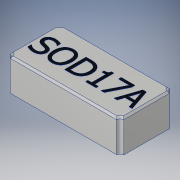
# Autodesk Inventor part: Crystal_ECX-34
Saved by Autodesk Inventor 2018 (Build 220112000, 112)
## iProperties
Created: 2016-08-15
Part Number: Crystal_ECX-34
Material: Aluminum 6061
Document SubType Name: Modeling
Designer: Bradley
Density: 2.7 g/cm^3
Appearance: Aluminum - Flat
Author: Bradley
Autodesk Inventor part; units mm, degrees
ref_plane "YZ Plane" through (0, 0, 0) normal (1, 0, 0) x (0, 1, 0)
ref_plane "XZ Plane" through (0, 0, 0) normal (0, 1, 0) x (-1, 0, 0)
ref_plane "XY Plane" through (0, 0, 0) normal (0, 0, 1) x (1, 0, 0)
sketch "Sketch1" plane through (0, 0, 0) normal (0, 1, 0) x (-1, 0, 0)
  line L0 (-1.6, 0.75) -> (1.6, 0.75)
  line L1 (1.6, 0.75) -> (1.6, -0.75)
  line L2 (1.6, -0.75) -> (-1.6, -0.75)
  line L3 (-1.6, -0.75) -> (-1.6, 0.75)
  line L4 (-1.6, 0.75) -> (1.6, -0.75) construction
  line L5 (1.6, 0.75) -> (-1.6, -0.75) construction
  arc A0 (1.6, -0.65) -> (1.5, -0.75) centre (1.6, -0.75) ccw
  arc A1 (-1.5, -0.75) -> (-1.6, -0.65) centre (-1.6, -0.75) ccw
  arc A2 (-1.6, 0.65) -> (-1.5, 0.75) centre (-1.6, 0.75) ccw
  arc A3 (1.5, 0.75) -> (1.6, 0.65) centre (1.6, 0.75) ccw
  point P0 (0, 0)
  dimension "d0" = 3.2
  dimension "d1" = 1.5
  dimension "d4" = 0.1
  constraints: 12 end point, 8 point on circle, 8 point on line, 4 centre point, 4 coincident, 3 equal radius, 2 midpoint, 2 parallel, 1 horizontal, 1 perpendicular
  measures "d0" distance of L1.end L2.end
  measures "d1" distance of L0.end L1.end
  measures "d4" radius of A0
extrude "Extrusion1" add sketch "Sketch1" along normal mid plane 0.9 contours L0 A3 L1 A0 L2 A1 L3 A2
chamfer "Chamfer1" distance 0.05 angle 45 8 edges at (0, 0.45, 0.75) (-1.5293, 0.45, 0.6793) (-1.6, 0.45, 0) (-1.5293, 0.45, -0.6793) (0, 0.45, -0.75) (1.5293, 0.45, -0.6793) (1.6, 0.45, 0) (1.5293, 0.45, 0.6793)
sketch "Sketch2" plane through (0, -0.45, 0) normal (0, -1, 0) x (1, 0, 0)
  line L0 (-1.6, 0.65) -> (-1.6, -0.65) projected
  arc A0 (-1.5, -0.75) -> (-1.6, -0.65) centre (-1.6, -0.75) ccw projected
  line L1 (-1.5, -0.75) -> (1.5, -0.75) projected
  arc A1 (1.6, -0.65) -> (1.5, -0.75) centre (1.6, -0.75) ccw projected
  line L2 (1.6, -0.65) -> (1.6, 0.65) projected
  arc A2 (1.5, 0.75) -> (1.6, 0.65) centre (1.6, 0.75) ccw projected
  line L3 (1.5, 0.75) -> (-1.5, 0.75) projected
  arc A3 (-1.6, 0.65) -> (-1.5, 0.75) centre (-1.6, 0.75) ccw projected
  arc A4 (-1.5, -0.75) -> (-1.6, -0.65) centre (-1.6, -0.75) ccw projected
  line L4 (-1.5741, -0.6534) -> (-1.5034, -0.5827)
  line L5 (-1.5034, -0.5827) -> (-1.5034, 0.5827)
  line L6 (-1.5034, 0.5827) -> (-1.5741, 0.6534)
  arc A5 (-1.6, 0.65) -> (-1.5, 0.75) centre (-1.6, 0.75) ccw projected
  line L7 (-1.5034, 0.7241) -> (-1.4327, 0.6534)
  line L8 (-1.4327, 0.6534) -> (-1.2, 0.6534)
  line L9 (-1.2, 0.6534) -> (-0.9, 0.3534)
  line L10 (-0.9, 0.3534) -> (-0.9, -0.6534)
  line L11 (-0.9, -0.6534) -> (-1.4327, -0.6534)
  line L12 (-1.4327, -0.6534) -> (-1.5034, -0.7241)
  arc A6 (1.5, 0.75) -> (1.6, 0.65) centre (1.6, 0.75) ccw projected
  line L13 (1.5034, 0.7241) -> (1.4327, 0.6534)
  line L14 (1.4327, 0.6534) -> (0.9, 0.6534)
  line L15 (0.9, 0.6534) -> (0.9, -0.6534)
  line L16 (0.9, -0.6534) -> (1.4327, -0.6534)
  line L17 (1.4327, -0.6534) -> (1.5034, -0.7241)
  arc A7 (1.6, -0.65) -> (1.5, -0.75) centre (1.6, -0.75) ccw projected
  line L18 (1.5741, -0.6534) -> (1.5034, -0.5827)
  line L19 (1.5034, -0.5827) -> (1.5034, 0.5827)
  line L20 (1.5034, 0.5827) -> (1.5741, 0.6534)
  line L21 (-1.6, 0.75) -> (-1.5293, 0.6793) construction
  line L22 (1.5, 0.75) -> (-1.5, 0.75) construction
  line L23 (-1.6, -0.75) -> (-1.5293, -0.6793) construction
  point P0 (0, 0)
  point P1 (0.9, 0)
  dimension "d8" = 1.8
  dimension "d9" = 0.1
  dimension "d10" = 0.3
  constraints: 38 end point, 15 point on circle, 9 equal length, 9 parallel, 7 perpendicular, 3 point on line, 1 collinear, 1 horizontal alignment, 1 midpoint, 1 vertical, 1 other
  measures "d8" distance between parallel lines of L15 L10
  measures "d9" distance between parallel lines of L6 L7
  measures "d10" horizontal distance of L8.end L9.end
extrude "Extrusion2" add sketch "Sketch2" along normal blind 0.01 contours A3 L7 L8 L9 L10 L11 L12 A0 L4 L5 L6 | A2 L20 L19 L18 A1 L17 L16 L15 L14 L13 | A2 L2 A1 L18 L19 L20
sketch "Sketch3" plane through (0, 0.45, 0) normal (0, 1, 0) x (1, 0, 0)
  line L0 (-1.4586, 0.7) -> (1.4586, 0.7) projected
  arc A0 (-1.55, 0.6086) -> (-1.4586, 0.7) centre (-1.6, 0.75) ccw projected
  line L1 (-1.55, -0.6086) -> (-1.55, 0.6086) projected
  arc A1 (-1.4586, -0.7) -> (-1.55, -0.6086) centre (-1.6, -0.75) ccw projected
  line L2 (1.4586, -0.7) -> (-1.4586, -0.7) projected
  arc A2 (1.55, -0.6086) -> (1.4586, -0.7) centre (1.6, -0.75) ccw projected
  line L3 (1.55, 0.6086) -> (1.55, -0.6086) projected
  arc A3 (1.4586, 0.7) -> (1.55, 0.6086) centre (1.6, 0.75) ccw projected
  line L4 (1.55, 0.6086) -> (1.55, -0.6086) construction
  line L5 (1.55, -0.3122) -> (-1.55, -0.3122) construction
  spline S0 degree 2 poles (-1.2751, -0.3229) (-1.3403, -0.3229) (-1.4317, -0.2957) (-1.472, -0.2762) knots 0 0 0 1 2 2 2
  line L6 (-1.472, -0.2762) -> (-1.472, -0.1761)
  line L7 (-1.472, -0.1761) -> (-1.4662, -0.1761)
  spline S1 degree 2 poles (-1.4662, -0.1761) (-1.4268, -0.213) (-1.3271, -0.2538) (-1.281, -0.2538) knots 0 0 0 1 2 2 2
  spline S2 degree 2 poles (-1.281, -0.2538) (-1.2148, -0.2538) (-1.1472, -0.1989) (-1.1472, -0.1537) knots 0 0 0 1 2 2 2
  spline S3 degree 2 poles (-1.1472, -0.1537) (-1.1472, -0.1177) (-1.1827, -0.073) (-1.2212, -0.0618) knots 0 0 0 1 2 2 2
  spline S4 degree 2 poles (-1.2212, -0.0618) (-1.2489, -0.054) (-1.2951, -0.0433) (-1.3296, -0.0346) knots 0 0 0 1 2 2 2
  spline S5 degree 2 poles (-1.3296, -0.0346) (-1.3607, -0.0263) (-1.4098, -0.0015) (-1.4288, 0.0184) knots 0 0 0 1 2 2 2
  spline S6 degree 2 poles (-1.4288, 0.0184) (-1.4472, 0.0384) (-1.4677, 0.0919) (-1.4677, 0.1269) knots 0 0 0 1 2 2 2
  spline S7 degree 2 poles (-1.4677, 0.1269) (-1.4677, 0.1998) (-1.3539, 0.2985) (-1.2659, 0.2985) knots 0 0 0 1 2 2 2
  spline S8 degree 2 poles (-1.2659, 0.2985) (-1.2153, 0.2985) (-1.1259, 0.2786) (-1.0874, 0.2596) knots 0 0 0 1 2 2 2
  line L8 (-1.0874, 0.2596) -> (-1.0874, 0.1643)
  line L9 (-1.0874, 0.1643) -> (-1.0933, 0.1643)
  spline S9 degree 2 poles (-1.0933, 0.1643) (-1.122, 0.1906) (-1.2114, 0.2295) (-1.2605, 0.2295) knots 0 0 0 1 2 2 2
  spline S10 degree 2 poles (-1.2605, 0.2295) (-1.316, 0.2295) (-1.3845, 0.1774) (-1.3845, 0.1351) knots 0 0 0 1 2 2 2
  spline S11 degree 2 poles (-1.3845, 0.1351) (-1.3845, 0.0972) (-1.3442, 0.052) (-1.3062, 0.0418) knots 0 0 0 1 2 2 2
  spline S12 degree 2 poles (-1.3062, 0.0418) (-1.281, 0.035) (-1.2075, 0.0175) (-1.1832, 0.0102) knots 0 0 0 1 2 2 2
  spline S13 degree 2 poles (-1.1832, 0.0102) (-1.1215, -0.0088) (-1.0641, -0.0851) (-1.0641, -0.141) knots 0 0 0 1 2 2 2
  spline S14 degree 2 poles (-1.0641, -0.141) (-1.0641, -0.1765) (-1.0928, -0.2446) (-1.1186, -0.2684) knots 0 0 0 1 2 2 2
  spline S15 degree 2 poles (-1.1186, -0.2684) (-1.1472, -0.2947) (-1.2202, -0.3229) (-1.2751, -0.3229) knots 0 0 0 1 2 2 2
  spline S16 degree 2 poles (-0.5584, 0.2192) (-0.5244, 0.1794) (-0.4865, 0.0627) (-0.4865, -0.0122) knots 0 0 0 1 2 2 2
  spline S17 degree 2 poles (-0.4865, -0.0122) (-0.4865, -0.0851) (-0.5234, -0.2033) (-0.5584, -0.2432) knots 0 0 0 1 2 2 2
  spline S18 degree 2 poles (-0.5584, -0.2432) (-0.5954, -0.285) (-0.6931, -0.3248) (-0.7519, -0.3248) knots 0 0 0 1 2 2 2
  spline S19 degree 2 poles (-0.7519, -0.3248) (-0.8127, -0.3248) (-0.91, -0.2835) (-0.9455, -0.2432) knots 0 0 0 1 2 2 2
  spline S20 degree 2 poles (-0.9455, -0.2432) (-0.98, -0.2033) (-1.0169, -0.0861) (-1.0169, -0.0122) knots 0 0 0 1 2 2 2
  spline S21 degree 2 poles (-1.0169, -0.0122) (-1.0169, 0.0632) (-0.9795, 0.1779) (-0.945, 0.2192) knots 0 0 0 1 2 2 2
  spline S22 degree 2 poles (-0.945, 0.2192) (-0.91, 0.2591) (-0.8122, 0.3004) (-0.7519, 0.3004) knots 0 0 0 1 2 2 2
  spline S23 degree 2 poles (-0.7519, 0.3004) (-0.6907, 0.3004) (-0.5925, 0.2577) (-0.5584, 0.2192) knots 0 0 0 1 2 2 2
  spline S24 degree 2 poles (-0.5696, -0.0122) (-0.5696, 0.0471) (-0.5954, 0.139) (-0.6187, 0.1692) knots 0 0 0 1 2 2 2
  spline S25 degree 2 poles (-0.6187, 0.1692) (-0.6425, 0.2003) (-0.7096, 0.2314) (-0.7515, 0.2314) knots 0 0 0 1 2 2 2
  spline S26 degree 2 poles (-0.7515, 0.2314) (-0.7947, 0.2314) (-0.8599, 0.2013) (-0.8847, 0.1692) knots 0 0 0 1 2 2 2
  spline S27 degree 2 poles (-0.8847, 0.1692) (-0.9085, 0.1385) (-0.9338, 0.0462) (-0.9338, -0.0122) knots 0 0 0 1 2 2 2
  spline S28 degree 2 poles (-0.9338, -0.0122) (-0.9338, -0.1303) (-0.8346, -0.2558) (-0.7515, -0.2558) knots 0 0 0 1 2 2 2
  spline S29 degree 2 poles (-0.7515, -0.2558) (-0.6683, -0.2558) (-0.5696, -0.1303) (-0.5696, -0.0122) knots 0 0 0 1 2 2 2
  spline S30 degree 2 poles (0.0741, -0.0127) (0.0741, -0.0949) (0.0075, -0.2271) (-0.0484, -0.2641) knots 0 0 0 1 2 2 2
  spline S31 degree 2 poles (-0.0484, -0.2641) (-0.0941, -0.2927) (-0.1879, -0.3122) (-0.2609, -0.3122) knots 0 0 0 1 2 2 2
  line L10 (-0.2609, -0.3122) -> (-0.3989, -0.3122)
  line L11 (-0.3989, -0.3122) -> (-0.3989, 0.2878)
  line L12 (-0.3989, 0.2878) -> (-0.2623, 0.2878)
  spline S32 degree 2 poles (-0.2623, 0.2878) (-0.1777, 0.2878) (-0.0814, 0.2625) (-0.0474, 0.2402) knots 0 0 0 1 2 2 2
  spline S33 degree 2 poles (-0.0474, 0.2402) (0.0105, 0.2017) (0.0741, 0.0748) (0.0741, -0.0127) knots 0 0 0 1 2 2 2
  spline S34 degree 2 poles (-0.009, -0.0117) (-0.009, 0.0573) (-0.0547, 0.1551) (-0.0999, 0.1828) knots 0 0 0 1 2 2 2
  spline S35 degree 2 poles (-0.0999, 0.1828) (-0.132, 0.2017) (-0.2045, 0.2188) (-0.2584, 0.2188) knots 0 0 0 1 2 2 2
  line L13 (-0.2584, 0.2188) -> (-0.3192, 0.2188)
  line L14 (-0.3192, 0.2188) -> (-0.3192, -0.2432)
  line L15 (-0.3192, -0.2432) -> (-0.2584, -0.2432)
  spline S36 degree 2 poles (-0.2584, -0.2432) (-0.2054, -0.2432) (-0.1252, -0.2261) (-0.0926, -0.2033) knots 0 0 0 1 2 2 2
  spline S37 degree 2 poles (-0.0926, -0.2033) (-0.0508, -0.1751) (-0.009, -0.0817) (-0.009, -0.0117) knots 0 0 0 1 2 2 2
  line L16 (0.4835, -0.3122) -> (0.1908, -0.3122)
  line L17 (0.1908, -0.3122) -> (0.1908, -0.2509)
  line L18 (0.1908, -0.2509) -> (0.2998, -0.2509)
  line L19 (0.2998, -0.2509) -> (0.2998, 0.1512)
  line L20 (0.2998, 0.1512) -> (0.1908, 0.1512)
  line L21 (0.1908, 0.1512) -> (0.1908, 0.2061)
  spline S38 degree 2 poles (0.1908, 0.2061) (0.2526, 0.2061) (0.3109, 0.2411) (0.3148, 0.2897) knots 0 0 0 1 2 2 2
  line L22 (0.3148, 0.2897) -> (0.3771, 0.2897)
  line L23 (0.3771, 0.2897) -> (0.3771, -0.2509)
  line L24 (0.3771, -0.2509) -> (0.4835, -0.2509)
  line L25 (0.4835, -0.2509) -> (0.4835, -0.3122)
  line L26 (0.9707, 0.1979) -> (0.7111, -0.3122)
  line L27 (0.7111, -0.3122) -> (0.6255, -0.3122)
  line L28 (0.6255, -0.3122) -> (0.8998, 0.2173)
  line L29 (0.8998, 0.2173) -> (0.59, 0.2173)
  line L30 (0.59, 0.2173) -> (0.59, 0.2878)
  line L31 (0.59, 0.2878) -> (0.9707, 0.2878)
  line L32 (0.9707, 0.2878) -> (0.9707, 0.1979)
  line L33 (0.9965, -0.3122) -> (1.1988, 0.2878)
  line L34 (1.1988, 0.2878) -> (1.297, 0.2878)
  line L35 (1.297, 0.2878) -> (1.4993, -0.3122)
  line L36 (1.4993, -0.3122) -> (1.4152, -0.3122)
  line L37 (1.4152, -0.3122) -> (1.3607, -0.1444)
  line L38 (1.3607, -0.1444) -> (1.1317, -0.1444)
  line L39 (1.1317, -0.1444) -> (1.0772, -0.3122)
  line L40 (1.0772, -0.3122) -> (0.9965, -0.3122)
  line L41 (1.3388, -0.0764) -> (1.2459, 0.2061)
  line L42 (1.2459, 0.2061) -> (1.1536, -0.0764)
  line L43 (1.1536, -0.0764) -> (1.3388, -0.0764)
  point P0 (0, 0)
  constraints: 2 end point, 2 point on line, 1 horizontal, 1 perpendicular
extrude "Extrusion3" add sketch "Sketch3" along normal blind 0.01 contours S0 L6 L7 S1 S2 S3 S4 S5 S6 S7 S8 L8 L9 S9 S10 S11 S12 S13 S14 S15 | S16 S17 S18 S19 S20 S21 S22 S23 | S30 S31 L10 L11 L12 S32 S33 | L16 L17 L18 L19 L20 L21 S38 L22 L23 L24 L25 | L26 L27 L28 L29 L30 L31 L32 | L33 L34 L35 L36 L37 L38 L39 L40
body "Solid1"
